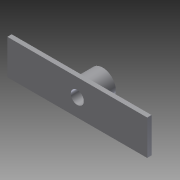
# Autodesk Inventor part: ferrous_insert
Saved by Autodesk Inventor 2011 (Build 150239000, 239)
## iProperties
Created: 2012-06-13
Part Number: ferrous_insert
Document SubType Name: Modeling
Designer: labuser
Density: 1 g/cm^3
Author: labuser
Autodesk Inventor part; units mm, degrees
ref_plane "YZ Plane" through (0, 0, 0) normal (1, 0, 0) x (0, 1, 0)
ref_plane "XZ Plane" through (0, 0, 0) normal (0, 1, 0) x (-1, 0, 0)
ref_plane "XY Plane" through (0, 0, 0) normal (0, 0, 1) x (1, 0, 0)
sketch "Sketch1" plane through (0, 0, 0) normal (0, 0, 1) x (1, 0, 0)
  circle A0 centre (0, 0) radius 4.75
  dimension "d0" = 9.5
  constraints: 1 centre point, 1 coincident
  measures "d0" diameter of A0
extrude "Extrusion1" add sketch "Sketch1" along normal blind 7.675
sketch "Sketch2" plane through (0, 0, 7.675) normal (0, 0, 1) x (1, 0, 0)
  circle A0 centre (0, 0) radius 4.75 projected
  circle A1 centre (0, 0) radius 2.3813
  dimension "d3" = 4.7625
  constraints: 1 centre point, 1 coincident
  measures "d3" diameter of A1
extrude "Extrusion2" cut sketch "Sketch2" against normal through all contours A1
sketch "Sketch3" plane through (0, 0, 7.675) normal (0, 0, 1) x (1, 0, 0)
  circle A0 centre (0, 0) radius 2.3813 projected
  line L0 (-25.4, -6.35) -> (25.4, -6.35)
  line L1 (25.4, -6.35) -> (25.4, 6.35)
  line L2 (25.4, 6.35) -> (-25.4, 6.35)
  line L3 (-25.4, 6.35) -> (-25.4, -6.35)
  dimension "d6" = 50.8
  dimension "d7" = 12.7
  constraints: 8 end point, 2 parallel, 1 horizontal, 1 perpendicular
  measures "d6" distance of L2.end L1.end
  measures "d7" distance of L1.end L0.end
extrude "Extrusion3" add sketch "Sketch3" along normal blind 1.5875
body "Solid1"
